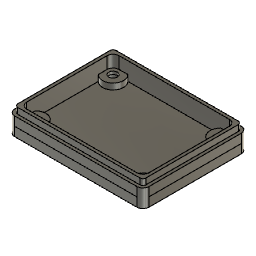
Base plug v2 (Autodesk Fusion 360 design; units mm, degrees)
Autodesk Fusion 360 part; units mm, degrees
sketch "Esquisse1" plane through (0, 0, 0) normal (0, 0, 1) x (1, 0, 0)
  line L0 (0, 0) -> (45, 0)
  line L1 (45, 0) -> (45, 35)
  line L2 (45, 35) -> (0, 35)
  line L3 (0, 35) -> (0, 0)
  circle A0 centre (2, 33) radius 2
  circle A1 centre (43, 33) radius 2
  circle A2 centre (43, 2) radius 2
  circle A3 centre (2, 2) radius 2
  line L4 (2, 33) -> (43, 33)
  line L5 (43, 33) -> (43, 2)
  line L6 (43, 2) -> (2, 2)
  line L7 (2, 2) -> (2, 33)
  dimension "d1" = 35
  dimension "d2" = 45
  constraint horizontal L0
  constraint vertical L1
  constraint horizontal L2
  constraint vertical L3
  constraint coincident L0.start L3.end
  constraint tangent L2 A0
  constraint tangent L2 A1
  constraint tangent L1 A2
  constraint tangent L0 A3
  constraint coincident A0.centre L4.start
  constraint coincident A1.centre L4.end
  constraint horizontal L4
  constraint coincident A2.centre L5.end
  constraint perpendicular L4 L5
  constraint coincident A3.centre L6.end
  constraint perpendicular L5 L6
  constraint perpendicular L4 L7
  measures "d1" distance of L0.start L2.end
  measures "d2" distance of L0.start L0.end
extrude "Extrusion1" add sketch "Esquisse1" along normal blind 3 contours L0 A2 A3 L6 | A3 L6 L7 | L3 A0 A3 L7 | A2 L5 L6 | A3 L6 L7 | A0 A1 A2 A3 L4 L5 L6 L7 | A0 L4 L7 | A2 L5 L6 | L1 A1 A2 L5 | L2 A0 A1 L4 | A0 L4 L7 | A1 L4 L5 | A1 L4 L5
sketch "Esquisse2" plane through (0, 0, 3) normal (0, 0, 1) x (-1, 0, 0)
  line L0 (0, -33) -> (0, -2)
  arc A0 (0, -2) -> (-2, 0) centre (-2, -2) ccw
  line L1 (-2, 0) -> (-43, 0)
  arc A1 (-43, 0) -> (-45, -2) centre (-43, -2) ccw
  line L2 (-45, -2) -> (-45, -33.0004)
  arc A2 (-45, -33.0004) -> (-43, -35) centre (-43, -33) ccw
  line L3 (-43, -35) -> (-2, -35)
  arc A3 (-2, -35) -> (0, -33) centre (-2, -33) ccw
  circle A4 centre (-4, -31) radius 2
  circle A5 centre (-4, -4) radius 2
  circle A6 centre (-41, -4) radius 2
  circle A7 centre (-41, -31) radius 2
  line L4 (-4, -33) -> (-41, -33)
  line L5 (-41, -2) -> (-4, -2)
  line L6 (-43, -4) -> (-43, -31)
  line L7 (-2, -31) -> (-2, -4)
  constraint coincident A4 L4.start
  constraint tangent A4 L4
  constraint parallel L3 L4
  constraint coincident A6 L5.start
  constraint coincident A5 L5.end
  constraint tangent A5 L5
  constraint coincident A6 L6.start
  constraint coincident A7 L6.end
  constraint tangent A7 L6
  constraint perpendicular L5 L6
  constraint coincident A4 L7.start
  constraint tangent A4 L7
  constraint vertical L7
extrude "Extrusion2" add sketch "Esquisse2" along normal blind 6
extrude "Extrusion3" cut 1 faces at (28.6667, 12.3333, 3) along direction (0, 0, -1) blind 1
sketch "Esquisse3" plane through (0, 0, 2) normal (0, 0, 1) x (-1, 0, 0)
  line L0 (-2, -31) -> (-2, -4)
  arc A0 (-2, -4) -> (-4, -2) centre (-4, -4) ccw
  line L1 (-4, -2) -> (-41, -2)
  arc A1 (-41, -2) -> (-43, -4) centre (-41, -4) ccw
  line L2 (-43, -4) -> (-43, -31)
  arc A2 (-43, -31) -> (-41, -33) centre (-41, -31) ccw
  line L3 (-41, -33) -> (-4, -33)
  arc A3 (-4, -33) -> (-2, -31) centre (-4, -31) ccw
  line L4 (-20, -2) -> (-20, -2.5)
  line L5 (-20, -33) -> (-20, -32.5)
  line L6 (-2, -15) -> (-2.5, -15)
  line L7 (-43, -17.5) -> (-42.5, -17.5)
  line L8 (-2, -11) -> (-2.5, -11)
  line L9 (-20, -32.5) -> (2.5659, -32.5)
  line L10 (2.5659, -32.5) -> (-53, -32.5)
  line L11 (-42.5, -17.5) -> (-42.5, -37)
  line L12 (-42.5, -37) -> (-42.5, 4)
  line L13 (-20, -2.5) -> (1, -2.5)
  line L14 (1, -2.5) -> (-48, -2.5)
  circle A4 centre (-4.5, -30.5) radius 2
  line L15 (-2.5, -11) -> (-2.5, -30.5)
  circle A5 centre (-4.5, -4.5) radius 2
  line L16 (-2.5, -4.4879) -> (-2.5, -15)
  circle A6 centre (-40, -4.5) radius 2
  circle A7 centre (-40.729, -4.5) radius 2
  dimension "d9" = 0.5
  dimension "d10" = 0.5
  dimension "d11" = 0.5
  dimension "d12" = 0.5
  dimension "d13" = 0.5
  constraint coincident L1 L4.start
  constraint perpendicular L1 L4
  constraint coincident L3 L5.start
  constraint perpendicular L3 L5
  constraint coincident L0 L6.start
  constraint perpendicular L0 L6
  constraint midpoint L2 L7.start
  constraint perpendicular L2 L7
  constraint coincident L0 L8.start
  constraint perpendicular L0 L8
  constraint perpendicular L5 L9
  constraint parallel L3 L10
  constraint perpendicular L10 L11
  constraint perpendicular L10 L12
  constraint perpendicular L4 L13
  constraint tangent L9 A4
  constraint coincident A4 L15.end
  constraint tangent A4 L15
  constraint perpendicular L8 L15
  constraint tangent L13 A5
  constraint tangent L14 A5
  constraint coincident A5 L16.start
  constraint tangent L14 A6
  constraint tangent L14 A7
  measures "d9" distance of L4.start L4.end
  measures "d10" distance of L5.start L5.end
  measures "d11" distance of L6.start L6.end
  measures "d12" distance of L7.start L7.end
  measures "d13" distance of L8.start L8.end
sketch "Esquisse4" plane through (0, 0, 2) normal (0, 0, 1) x (1, 0, 0)
  line L0 (42.5, 4.5) -> (40.5, 4.5)
  circle A0 centre (40.5, 4.5) radius 2
  circle A1 centre (40.5, 30.5) radius 2.0147
  circle A2 centre (4.5, 30.5) radius 3.5
  circle A3 centre (4.5, 4.5) radius 3.5
  circle A4 centre (40.5, 4.5) radius 3.5
  circle A5 centre (40.5, 30.5) radius 3.5
  circle A6 centre (4, 31) radius 2
  circle A7 centre (41, 31) radius 2
  circle A8 centre (41, 4) radius 2
  circle A9 centre (4, 4) radius 2
  line L1 (2.0023, 28.0482) -> (2, 30.9984)
  line L2 (6.9527, 32.9969) -> (4.0021, 33)
  line L3 (38.0505, 33) -> (40.89, 32.997)
  line L4 (42.9978, 28.0483) -> (43, 30.9985)
  line L5 (43, 6.9495) -> (43, 4)
  line L6 (38.0503, 2.0002) -> (40.9999, 2)
  line L7 (6.949, 1.9995) -> (3.9997, 2)
  line L8 (2.0005, 6.95) -> (2, 4.0004)
  dimension "d14" = 2
  dimension "d15" = 7
  dimension "d16" = 7
  dimension "d17" = 7
  dimension "d18" = 7
  dimension "d19" = 4
  dimension "d20" = 4
  dimension "d21" = 4
  dimension "d22" = 4
  constraint horizontal L0
  constraint coincident L0.end A0.centre
  constraint coincident L0.start A0
  constraint coincident A2 L1.start
  constraint coincident A6 L1.end
  constraint tangent A6 L1
  constraint coincident A2 L2.start
  constraint coincident A6 L2.end
  constraint tangent A6 L2
  constraint coincident A5 L3.start
  constraint coincident A7 L3.end
  constraint parallel L2 L3
  constraint coincident A5 L4.start
  constraint coincident A7 L4.end
  constraint tangent A7 L4
  constraint coincident A4 L5.start
  constraint coincident A8 L5.end
  constraint tangent A8 L5
  constraint coincident A4 L6.start
  constraint coincident A8 L6.end
  constraint tangent A8 L6
  constraint coincident A3 L7.start
  constraint coincident A9 L7.end
  constraint tangent A9 L7
  constraint coincident A3 L8.start
  constraint coincident A9 L8.end
  constraint tangent A9 L8
  measures "d14" distance of L0.start L0.end
  measures "d15" diameter of A2
  measures "d16" diameter of A3
  measures "d17" diameter of A4
  measures "d18" diameter of A5
  measures "d19" diameter of A6
  measures "d20" diameter of A7
  measures "d21" diameter of A8
  measures "d22" diameter of A9
extrude "Extrusion4" add sketch "Esquisse4" along normal blind 2 contours A0 A8 | A0 A8 | A0 A8 | A0 A4 A8 L5 L6 | A1 A7 | A1 A7 | A1 A7 | A1 A5 A7 L3 L4 | A2 A6 L1 L2 | A6 | A3 A9 L7 L8 | A9 picked at (6.0818, 28.238) picked at (6.0812, 6.7624)
sketch "Esquisse5" plane through (0, 0, 4) normal (0, 0, 1) x (-1, 0, 0)
  arc A0 (-2.0023, -28.0482) -> (-6.9527, -32.9969) centre (-4.5, -30.5) ccw
  line L0 (-6.9527, -32.9969) -> (-4.0021, -33)
  line L1 (-4.0021, -33) -> (-4, -33)
  arc A1 (-4, -33) -> (-2, -31) centre (-4, -31) ccw
  line L2 (-2, -31) -> (-2, -30.9984)
  line L3 (-2, -30.9984) -> (-2.0023, -28.0482)
  line L4 (-42.5, -30.5) -> (-40.5, -30.5)
  line L5 (-2.5, -4.5) -> (-4.5, -4.5016)
  circle A2 centre (-4.5, -30.5) radius 1.45
  circle A3 centre (-40.5, -30.5) radius 1.45
  circle A4 centre (-4.5, -4.5016) radius 1.45
  circle A5 centre (-40.5, -4.5) radius 1.45
  dimension "d27" = 38
  dimension "d28" = 2
  dimension "d29" = 2.9
  dimension "d30" = 2.9
  dimension "d31" = 2.9
  dimension "d32" = 2.9
  constraint perpendicular L3 L5
  constraint coincident L4.end A3.centre
  constraint coincident L5.end A4.centre
  measures "d27" distance of L5.start A5.centre
  measures "d28" distance of L5.start L5.end
  measures "d29" diameter of A2
  measures "d30" diameter of A3
  measures "d31" diameter of A4
  measures "d32" diameter of A5
extrude "Extrusion5" cut sketch "Esquisse5" against normal blind 10 contours A2 | A3 | A4 | A5
sketch "Esquisse6" plane through (0, 0, 0) normal (0, 0, -1) x (1, 0, 0)
  circle A0 centre (40.5, -30.5) radius 1.45
  circle A1 centre (4.5, -4.5016) radius 1.45
  circle A2 centre (4.5, -30.5) radius 1.45
  circle A3 centre (40.5, -4.5) radius 1.45
  line L0 (0, -2) -> (0, -33)
  arc A4 (0, -33) -> (2, -35) centre (2, -33) ccw
  line L1 (2, -35) -> (43, -35)
  arc A5 (43, -35) -> (45, -33.0004) centre (43, -33) ccw
  line L2 (45, -33.0004) -> (45, -2)
  arc A6 (45, -2) -> (43, 0) centre (43, -2) ccw
  line L3 (43, 0) -> (2, 0)
  arc A7 (2, 0) -> (0, -2) centre (2, -2) ccw
  circle A8 centre (4.5, -4.5016) radius 2.5
  circle A9 centre (40.5, -4.5) radius 2.5
  circle A10 centre (4.5, -30.5) radius 2.5
  circle A11 centre (40.5, -30.5) radius 2.5
  dimension "d35" = 5
  dimension "d36" = 5
  dimension "d37" = 5
  dimension "d38" = 5
  constraint concentric A1 A8
  constraint concentric A3 A9
  constraint concentric A2 A10
  constraint concentric A0 A11
  measures "d35" diameter of A8
  measures "d36" diameter of A9
  measures "d37" diameter of A10
  measures "d38" diameter of A11
extrude "Extrusion6" cut sketch "Esquisse6" against normal blind 3 contours A8 | A9 | A10 | A11
sketch "Esquisse7" plane through (0, 0, 9) normal (0, 0, 1) x (-1, 0, 0)
  arc A0 (-4, -33) -> (-2, -31) centre (-4, -31) ccw
  line L0 (-4, -33) -> (-41, -33)
  arc A1 (-43, -31) -> (-41, -33) centre (-41, -31) ccw
  line L1 (-43, -31) -> (-43, -4)
  arc A2 (-41, -2) -> (-43, -4) centre (-41, -4) ccw
  line L2 (-41, -2) -> (-4, -2)
  arc A3 (-2, -4) -> (-4, -2) centre (-4, -4) ccw
  line L3 (-2, -4) -> (-2, -31)
  arc A4 (-2, -35) -> (0, -33) centre (-2, -33) ccw
  line L4 (0, -33) -> (0, -2)
  arc A5 (0, -2) -> (-2, 0) centre (-2, -2) ccw
  line L5 (-2, 0) -> (-43, 0)
  arc A6 (-43, 0) -> (-45, -2) centre (-43, -2) ccw
  line L6 (-45, -2) -> (-45, -33.0004)
  arc A7 (-45, -33.0004) -> (-43, -35) centre (-43, -33) ccw
  line L7 (-43, -35) -> (-2, -35)
extrude "Extrusion7" cut sketch "Esquisse7" against normal blind 1
sketch "Esquisse8" plane through (0, 0, 8) normal (0, 0, 1) x (-1, 0, 0)
  arc A0 (-41, -2) -> (-43, -4) centre (-41, -4) ccw
  line L0 (-41, -2) -> (-4, -2)
  arc A1 (-2, -4) -> (-4, -2) centre (-4, -4) ccw
  line L1 (-2, -4) -> (-2, -31)
  arc A2 (-4, -33) -> (-2, -31) centre (-4, -31) ccw
  line L2 (-4, -33) -> (-41, -33)
  arc A3 (-43, -31) -> (-41, -33) centre (-41, -31) ccw
  line L3 (-43, -31) -> (-43, -4)
  line L4 (-43, -35) -> (-2, -35)
  arc A4 (-2, -35) -> (0, -33) centre (-2, -33) ccw
  line L5 (0, -33) -> (0, -2)
  arc A5 (0, -2) -> (-2, 0) centre (-2, -2) ccw
  line L6 (-2, 0) -> (-43, 0)
  arc A6 (-43, 0) -> (-45, -2) centre (-43, -2) ccw
  line L7 (-45, -2) -> (-45, -33.0004)
  arc A7 (-45, -33.0004) -> (-43, -35) centre (-43, -33) ccw
  line L8 (-2, -1) -> (-43, -1)
  line L9 (-2, -34) -> (-43, -34)
  line L10 (-44, -33) -> (-44, -2)
  line L11 (-1, -33) -> (-1, -2)
  circle A8 centre (-2, -2) radius 1
  circle A9 centre (-2, -33) radius 1
  circle A10 centre (-43, -33) radius 1
  circle A11 centre (-43, -2) radius 1
  constraint perpendicular L1 L8
  constraint parallel L4 L9
  constraint parallel L7 L10
  constraint parallel L5 L11
  constraint concentric A5 A8
  constraint coincident L8.start A8
  constraint tangent L8 A8
  constraint concentric A4 A9
  constraint coincident L9.start A9
  constraint tangent L9 A9
  constraint concentric A7 A10
  constraint coincident L10.start A10
  constraint concentric A6 A11
  constraint coincident L10.end A11
extrude "Extrusion8" cut sketch "Esquisse8" against normal blind 2
